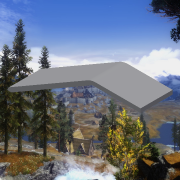
# Autodesk Inventor part: C14_TK_SlamRampConcept
Saved by Autodesk Inventor 2015 SP1 (Build 190203100, 203)
## iProperties
Created: 2016-01-19
Part Number: C14_TK_SlamRampConcept
Material: Generic
Document SubType Name: Modeling
Designer: TheeTimatahee
Density: 1 g/cm^3
Appearance: Default
Author: TheeTimatahee
Autodesk Inventor part; units mm, degrees
ref_plane "YZ Plane" through (0, 0, 0) normal (1, 0, 0) x (0, 1, 0)
ref_plane "XZ Plane" through (0, 0, 0) normal (0, 1, 0) x (-1, 0, 0)
ref_plane "XY Plane" through (0, 0, 0) normal (0, 0, 1) x (1, 0, 0)
sketch "Sketch1" plane through (0, 0, 0) normal (0, 0, 1) x (1, 0, 0)
  line L0 (-1.5983, -6.4434) -> (1.5767, -6.4434)
  line L1 (1.5767, -6.4434) -> (65.6988, 30.5775)
  line L2 (65.6988, 30.5775) -> (103.7988, 30.5775)
  line L3 (103.7988, 30.5775) -> (103.7988, 33.7525)
  line L4 (103.7988, 33.7525) -> (68.251, 33.7525)
  line L5 (-1.5983, -6.4434) -> (-1.5983, -6.4434)
  line L6 (-0.0108, -3.6937) -> (61.901, 32.0511)
  arc A0 (-0.0108, -3.6937) -> (-1.5983, -6.4434) centre (1.5767, -6.4434) ccw
  arc A1 (68.251, 33.7525) -> (61.901, 32.0511) centre (68.251, 21.0525) ccw
  dimension "d0" = 3.175
  dimension "d1" = 150
  dimension "d2" = 74.0418
  dimension "d3" = 38.1
  dimension "d5" = 3.175
  dimension "d6" = 3.175
  dimension "d7" = 3.175
  dimension "d8" = 12.7
  constraints: 14 end point, 4 point on circle, 4 tangent, 2 centre point, 2 horizontal, 2 vertical, 1 parallel, 1 perpendicular
  measures "d0" distance of L0.start L0.end
  measures "d1" angle of L0 L1
  measures "d2" distance of L0.end L1.end
  measures "d3" distance of L1.end L2.end
  measures "d5" distance between parallel lines of L6 L1
  measures "d6" distance of L2.end L3.end
  measures "d7" radius of A0
  measures "d8" radius of A1
extrude "Extrusion1" add sketch "Sketch1" along normal blind 25.4
sketch "Sketch2" plane through (68.251, 33.7525, 0) normal (0, 1, 0) x (1, 0, 0)
  line L0 (269.8757, -21.59) -> (269.8757, -12.7762) projected
  line L1 (252.8944, -12.7762) -> (269.8757, -12.7762) projected
  line L2 (227.4944, -12.7762) -> (248.757, -12.7762) projected
  line L3 (202.0944, -12.7762) -> (223.357, -12.7762) projected
  line L4 (176.6944, -12.7762) -> (197.957, -12.7762) projected
  line L5 (151.2944, -12.7762) -> (172.557, -12.7762) projected
  line L6 (125.8944, -12.7762) -> (147.157, -12.7762) projected
  line L7 (100.4944, -12.7762) -> (121.757, -12.7762) projected
  line L8 (75.0944, -12.7762) -> (96.357, -12.7762) projected
  line L9 (49.6944, -12.7762) -> (70.957, -12.7762) projected
  line L10 (24.2944, -12.7762) -> (45.557, -12.7762) projected
  line L11 (-1.1056, -12.7762) -> (20.157, -12.7762) projected
  line L12 (-22.8122, -12.7762) -> (-22.8122, -25.4) projected
  line L13 (-22.8122, -25.4) -> (676.8636, -25.4) projected
  line L14 (676.8636, -25.4) -> (676.8636, -12.7762) projected
  line L15 (633.8944, -12.7762) -> (655.157, -12.7762) projected
  line L16 (608.4944, -12.7762) -> (629.757, -12.7762) projected
  line L17 (583.0944, -12.7762) -> (604.357, -12.7762) projected
  line L18 (557.6944, -12.7762) -> (578.957, -12.7762) projected
  line L19 (532.2944, -12.7762) -> (553.557, -12.7762) projected
  line L20 (506.8944, -12.7762) -> (528.157, -12.7762) projected
  line L21 (481.4944, -12.7762) -> (502.757, -12.7762) projected
  line L22 (456.0944, -12.7762) -> (477.357, -12.7762) projected
  line L23 (430.6944, -12.7762) -> (451.957, -12.7762) projected
  line L24 (405.2944, -12.7762) -> (426.557, -12.7762) projected
  line L25 (384.1757, -12.7762) -> (401.157, -12.7762) projected
  line L26 (384.1757, -12.7762) -> (384.1757, -21.59) projected
  line L27 (384.1757, -21.59) -> (269.8757, -21.59) projected
  line L28 (-22.8122, -12.7762) -> (-5.243, -12.7762) projected
  line L29 (659.2944, -12.7762) -> (676.8636, -12.7762) projected
  arc A0 (248.757, -12.7762) -> (252.8944, -12.7762) centre (250.8257, -12.7) ccw projected
  arc A1 (223.357, -12.7762) -> (227.4944, -12.7762) centre (225.4257, -12.7) ccw projected
  arc A2 (197.957, -12.7762) -> (202.0944, -12.7762) centre (200.0257, -12.7) ccw projected
  arc A3 (172.557, -12.7762) -> (176.6944, -12.7762) centre (174.6257, -12.7) ccw projected
  arc A4 (147.157, -12.7762) -> (151.2944, -12.7762) centre (149.2257, -12.7) ccw projected
  arc A5 (121.757, -12.7762) -> (125.8944, -12.7762) centre (123.8257, -12.7) ccw projected
  arc A6 (96.357, -12.7762) -> (100.4944, -12.7762) centre (98.4257, -12.7) ccw projected
  arc A7 (70.957, -12.7762) -> (75.0944, -12.7762) centre (73.0257, -12.7) ccw projected
  arc A8 (45.557, -12.7762) -> (49.6944, -12.7762) centre (47.6257, -12.7) ccw projected
  arc A9 (20.157, -12.7762) -> (24.2944, -12.7762) centre (22.2257, -12.7) ccw projected
  arc A10 (629.757, -12.7762) -> (633.8944, -12.7762) centre (631.8257, -12.7) ccw projected
  arc A11 (604.357, -12.7762) -> (608.4944, -12.7762) centre (606.4257, -12.7) ccw projected
  arc A12 (578.957, -12.7762) -> (583.0944, -12.7762) centre (581.0257, -12.7) ccw projected
  arc A13 (553.557, -12.7762) -> (557.6944, -12.7762) centre (555.6257, -12.7) ccw projected
  arc A14 (528.157, -12.7762) -> (532.2944, -12.7762) centre (530.2257, -12.7) ccw projected
  arc A15 (502.757, -12.7762) -> (506.8944, -12.7762) centre (504.8257, -12.7) ccw projected
  arc A16 (477.357, -12.7762) -> (481.4944, -12.7762) centre (479.4257, -12.7) ccw projected
  arc A17 (451.957, -12.7762) -> (456.0944, -12.7762) centre (454.0257, -12.7) ccw projected
  arc A18 (426.557, -12.7762) -> (430.6944, -12.7762) centre (428.6257, -12.7) ccw projected
  arc A19 (401.157, -12.7762) -> (405.2944, -12.7762) centre (403.2257, -12.7) ccw projected
  arc A20 (-5.243, -12.7762) -> (-1.1056, -12.7762) centre (-3.1743, -12.7) ccw projected
  arc A21 (655.157, -12.7762) -> (659.2944, -12.7762) centre (657.2257, -12.7) ccw projected
  point P0 (-68.251, 0)
hole "Hole1" [suppressed]
body "Solid1"
